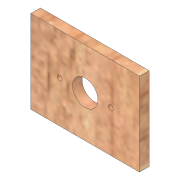
# Autodesk Inventor part: Firewall
Saved by Autodesk Inventor 2019 (Build 230136000, 136)
## iProperties
Created: 2022-04-02
Part Number: Firewall
Material: Plywood
Document SubType Name: Modeling
Designer: solyo
Density: 0.746667 g/cm^3
Appearance: Birch - Natural Polished
Mass: 1.85965 g
Surface Area: 21.2407 cm^2
Volume: 2.4906 cm^3
Author: solyo
Autodesk Inventor part; units mm, degrees
ref_plane "YZ Plane" through (0, 0, 0) normal (1, 0, 0) x (0, 1, 0)
ref_plane "XZ Plane" through (0, 0, 0) normal (0, 1, 0) x (-1, 0, 0)
ref_plane "XY Plane" through (0, 0, 0) normal (0, 0, 1) x (1, 0, 0)
sketch "Sketch1" plane through (0, 0, 0) normal (0, 0, 1) x (1, 0, 0)
  line L0 (17, -13) -> (-17, -13)
  line L1 (-17, -13) -> (-17, 13)
  line L2 (-17, 13) -> (17, 13)
  line L3 (17, 13) -> (17, -13)
  line L4 (17, -13) -> (-17, 13) construction
  line L5 (-17, -13) -> (17, 13) construction
  point P0 (0, 0)
  dimension "d0" = 34
  dimension "d1" = 26
  constraints: 12 end point, 2 midpoint, 2 parallel, 1 horizontal, 1 perpendicular
  measures "d0" distance of L1.end L2.end
  measures "d1" distance of L0.end L1.end
extrude "Extrusion1" add sketch "Sketch1" along normal blind 3
sketch "Sketch3" plane through (0, 0, 3) normal (0, 0, 1) x (1, 0, 0)
  point P0 (0, 0)
  point P1 (-8, 0)
  point P2 (8, 0)
  point P3 (0, 6)
  point P4 (0, -6)
  dimension "d4" = 12
  dimension "d5" = 16
  dimension "d6" = 8
  dimension "d7" = 6
  constraints: 2 horizontal alignment, 2 vertical alignment
  measures "d4" distance of point (0, -6) point (0, 6)
  measures "d5" distance of point (-8, 0) point (8, 0)
  measures "d6" distance of point (0, 0) point (-8, 0)
  measures "d7" distance of point (0, 0) point (0, 6)
hole "Hole1" at (-8, 0, 3) at (8, 0, 3) direction (0, 0, -1) diameter 1.5 end through all
sketch "Sketch4" plane through (0, 0, 3) normal (0, 0, 1) x (1, 0, 0)
  point P0 (0, 0)
  point P1 (0, 0)
  constraints: 1 coincident
hole "Hole2" at (0, 0, 3) direction (0, 0, -1) diameter 8 end through all
equation "\"d6\" = 0.5 * d5"
equation "\"d7\" = 0.5 * d4"
body "Solid1"
